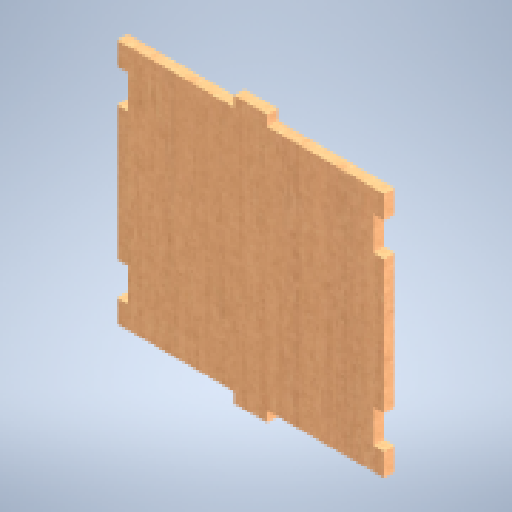
# Autodesk Inventor part: Left Panel
Saved by Autodesk Inventor 2023.1 (Build 271208000, 208)
## iProperties
Created: 2022-07-14
Part Number: Left Panel
Material: Wood (Cherry)
Document SubType Name: Modeling
Designer: Eli
Density: 0.63 g/cm^3
Appearance: Cherry - Natural Low Gloss
Author: Eli
Autodesk Inventor part; units mm, degrees
ref_plane "YZ Plane" through (0, 0, 0) normal (1, 0, 0) x (0, 1, 0)
ref_plane "XZ Plane" through (0, 0, 0) normal (0, 1, 0) x (-1, 0, 0)
ref_plane "XY Plane" through (0, 0, 0) normal (0, 0, 1) x (1, 0, 0)
sketch "Sketch1" plane through (0, 0, 0) normal (0, 0, 1) x (1, 0, 0)
  line L0 (0, 0) -> (0, -50.8) projected
  line L1 (0, -50.8) -> (4, -50.8) projected
  line L2 (4, 0) -> (4, -50.8) projected
  line L3 (0, 0) -> (4, 0) projected
  line L4 (0, -63.5) -> (0, -72.2) projected
  line L5 (0, -72.2) -> (4, -72.2) projected
  line L6 (4, -63.5) -> (4, -72.2) projected
  line L7 (0, -63.5) -> (4, -63.5) projected
  line L8 (0, 21.4) -> (0, 12.7) projected
  line L9 (0, 12.7) -> (4, 12.7) projected
  line L10 (4, 21.4) -> (4, 12.7) projected
  line L11 (0, 21.4) -> (4, 21.4) projected
  line L12 (44.45, 25.4) -> (57.15, 25.4) projected
  line L13 (44.45, 25.4) -> (44.45, 21.4) projected
  line L14 (44.45, 21.4) -> (57.15, 21.4) projected
  line L15 (57.15, 25.4) -> (57.15, 21.4) projected
  line L16 (44.45, -76.2) -> (57.15, -76.2) projected
  line L17 (57.15, -76.2) -> (57.15, -72.2) projected
  line L18 (44.45, -72.2) -> (57.15, -72.2) projected
  line L19 (44.45, -76.2) -> (44.45, -72.2) projected
  line L20 (101.6, 21.4) -> (4, 21.4)
  line L21 (4, 21.4) -> (4, -72.2)
  line L22 (4, -72.2) -> (101.6, -72.2)
  line L23 (101.6, -72.2) -> (101.6, 21.4)
  line L24 (50.8, 21.4) -> (50.8, -72.2)
  line L25 (101.6, 0) -> (101.6, -50.8)
  line L26 (101.6, -50.8) -> (97.6, -50.8)
  line L27 (97.6, 0) -> (97.6, -50.8)
  line L28 (101.6, 0) -> (97.6, 0)
  line L29 (101.6, -63.5) -> (101.6, -72.2)
  line L30 (101.6, -72.2) -> (97.6, -72.2)
  line L31 (97.6, -63.5) -> (97.6, -72.2)
  line L32 (101.6, -63.5) -> (97.6, -63.5)
  line L33 (101.6, 21.4) -> (101.6, 12.7)
  line L34 (101.6, 12.7) -> (97.6, 12.7)
  line L35 (101.6, 21.4) -> (97.6, 21.4)
  line L36 (97.6, 12.7) -> (97.6, 21.4)
  line L37 (97.6, 12.7) -> (97.6, 0)
  line L38 (97.6, -50.8) -> (97.6, -63.5)
  constraints: 38 end point, 10 symmetric about line, 3 equal length, 3 perpendicular, 2 point on line, 1 coincident, 1 horizontal, 1 vertical, 1 other
extrude "Extrusion1" add sketch "Sketch1" along normal blind 4 contours L3 L2 L1 L0 | L21 L10 L20 L14 L24 L18 L22 L6 L2 | L9 L8 L11 L10 | L6 L5 L4 L7 | L13 L12 L15 L14 | L18 L17 L16 L19 | L14 L20 L36 L37 L27 L38 L31 L22 L18 L24 | L20 L23 L34 L36 | L31 L32 L23 L22 | L28 L23 L26 L27
ref_plane "Work Plane1" through (50.8, -50.8, 0) normal (1, 0, 0) x (0, 0, -1)
sketch "Sketch2" plane through (0, 0, 4) normal (0, 0, 1) x (1, 0, 0)
  circle A0 centre (10.35, 6.35) radius 1.905
  line L0 (4, 12.7) -> (4, 0) projected
  point P0 (0, 0)
  point P1 (4, 6.35)
  point P2 (4, 6.35)
  dimension "d2" = 3.81
  dimension "d3" = 6.35
  constraints: 2 midpoint, 1 centre point, 1 horizontal alignment
  measures "d2" diameter of A0
  measures "d3" distance of point (4, 6.35) A0.centre
extrude "Extrusion2" cut sketch "Sketch2" against normal through all
body "Solid1"
